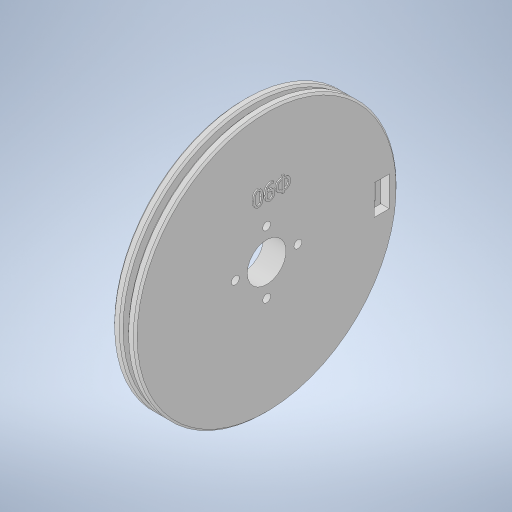
# Autodesk Inventor part: pully_shoulder2_90
Saved by Autodesk Inventor 2024 (Build 280153000, 153)
## iProperties
Created: 2025-06-10
Part Number: pully_shoulder2_90
Material: 一般
Document SubType Name: Modeling
Designer: HosodaLab2
Density: 1 g/cm^3
Appearance: 既定
Author: HosodaLab2
Autodesk Inventor part; units mm, degrees
ref_plane "YZ Plane" through (0, 0, 0) normal (1, 0, 0) x (0, 1, 0)
ref_plane "XZ Plane" through (0, 0, 0) normal (0, 1, 0) x (-1, 0, 0)
ref_plane "XY Plane" through (0, 0, 0) normal (0, 0, 1) x (1, 0, 0)
sketch "スケッチ1" plane through (0, 0, 0) normal (0, 1, 0) x (-1, 0, 0)
  circle A0 centre (0, 0) radius 45
  dimension "d0" = 90
  constraints: 1 centre point, 1 coincident
  measures "d0" diameter of A0
extrude "押し出し1" add sketch "スケッチ1" along normal blind 2.2
sketch "スケッチ2" plane through (0, 2.2, 0) normal (0, 1, 0) x (1, 0, 0)
  circle A0 centre (0, 0) radius 52.5
  line L0 (-4.0726, -27.1836) -> (5.4532, -27.1836) construction
  line L1 (5.4532, -27.1836) -> (5.4532, -31.1043) construction
  line L2 (5.4532, -31.1043) -> (-4.0726, -31.1043) construction
  line L3 (-4.0726, -31.1043) -> (-4.0726, -27.1836) construction
  dimension "d3" = 105
  constraints: 1 centre point, 1 coincident, 2 other
  measures "d3" diameter of A0
extrude "押し出し2" add sketch "スケッチ2" along normal blind 3.4
chamfer "面取り1" distance 0.75 angle 45 1 edges at (-52.5, 2.2, 0)
chamfer "面取り2" distance 0.75 angle 45 1 edges at (-52.5, 5.6, 0)
sketch "スケッチ3" plane through (0, 0, 0) normal (0, -1, 0) x (1, 0, 0)
  circle A0 centre (0, 0) radius 52.5
  dimension "d12" = 105
  constraints: 1 centre point, 1 coincident
  measures "d12" diameter of A0
extrude "押し出し3" add sketch "スケッチ3" along normal blind 3.4
chamfer "面取り3" distance 0.75 angle 45 1 edges at (-52.5, 0, 0)
chamfer "面取り4" distance 0.75 angle 45 1 edges at (-52.5, -3.4, 0)
sketch "スケッチ6" plane through (0, 5.6, 0) normal (0, 1, 0) x (1, 0, 0)
  circle A0 centre (0, 0) radius 7.65
  line L0 (0, 7.65) -> (46.8799, 7.65)
  circle A1 centre (0, 0) radius 47.5 projected
  line L1 (0, -7.65) -> (46.8799, -7.65)
  dimension "d39" = 15.3
  constraints: 4 end point, 4 point on circle, 1 centre point, 1 coincident, 1 horizontal, 1 parallel, 1 tangent
  measures "d39" diameter of A0
extrude "押し出し5" [suppressed]
chamfer "面取り7" [suppressed]
chamfer "面取り8" [suppressed]
chamfer "面取り9" [suppressed]
sketch "スケッチ7" plane through (0, 5.6, 0) normal (0, 1, 0) x (1, 0, 0)
  line L0 (-9.3358, -20.9354) -> (21.308, -20.9354) construction
  line L1 (21.308, -20.9354) -> (21.308, -27.5341) construction
  line L2 (21.308, -27.5341) -> (-9.3358, -27.5341) construction
  line L3 (-9.3358, -27.5341) -> (-9.3358, -20.9354) construction
  spline S0 degree 2 poles (-5.7914, -21.6571) (-5.2131, -21.667) (-4.2541, -22.0526) (-3.9377, -22.3739) knots 0 0 0 1 2 2 2
  spline S1 degree 2 poles (-3.9377, -22.3739) (-3.646, -22.6754) (-3.3247, -23.5207) (-3.3247, -24.0645) knots 0 0 0 1 2 2 2
  spline S2 degree 2 poles (-3.3247, -24.0645) (-3.3247, -24.633) (-3.6708, -25.5079) (-3.9772, -25.8045) knots 0 0 0 1 2 2 2
  spline S3 degree 2 poles (-3.9772, -25.8045) (-4.3084, -26.1308) (-5.2773, -26.4916) (-5.7914, -26.5015) knots 0 0 0 1 2 2 2
  line L4 (-5.7914, -26.5015) -> (-5.7914, -27.2084)
  line L5 (-5.7914, -27.2084) -> (-6.6021, -27.2084)
  line L6 (-6.6021, -27.2084) -> (-6.6021, -26.5015)
  spline S4 degree 2 poles (-6.6021, -26.5015) (-7.1162, -26.4867) (-8.0802, -26.1506) (-8.4213, -25.8144) knots 0 0 0 1 2 2 2
  spline S5 degree 2 poles (-8.4213, -25.8144) (-8.7277, -25.5129) (-9.0688, -24.628) (-9.0688, -24.0645) knots 0 0 0 1 2 2 2
  spline S6 degree 2 poles (-9.0688, -24.0645) (-9.0688, -23.5306) (-8.7426, -22.6853) (-8.446, -22.3788) knots 0 0 0 1 2 2 2
  spline S7 degree 2 poles (-8.446, -22.3788) (-8.1296, -22.0526) (-7.1805, -21.672) (-6.6021, -21.6571) knots 0 0 0 1 2 2 2
  line L7 (-6.6021, -21.6571) -> (-6.6021, -21.0096)
  line L8 (-6.6021, -21.0096) -> (-5.7914, -21.0096)
  line L9 (-5.7914, -21.0096) -> (-5.7914, -21.6571)
  spline S8 degree 2 poles (-5.7914, -25.8886) (-5.4207, -25.8787) (-4.8473, -25.6562) (-4.6594, -25.4684) knots 0 0 0 1 2 2 2
  spline S9 degree 2 poles (-4.6594, -25.4684) (-4.4073, -25.2212) (-4.17, -24.5143) (-4.17, -24.0299) knots 0 0 0 1 2 2 2
  spline S10 degree 2 poles (-4.17, -24.0299) (-4.17, -23.6245) (-4.3974, -22.9572) (-4.6248, -22.7249) knots 0 0 0 1 2 2 2
  spline S11 degree 2 poles (-4.6248, -22.7249) (-4.8374, -22.5024) (-5.4009, -22.2899) (-5.7914, -22.28) knots 0 0 0 1 2 2 2
  line L10 (-5.7914, -22.28) -> (-5.7914, -25.8886)
  spline S12 degree 2 poles (-6.6021, -22.28) (-6.9926, -22.2849) (-7.5562, -22.5074) (-7.7687, -22.7249) knots 0 0 0 1 2 2 2
  spline S13 degree 2 poles (-7.7687, -22.7249) (-7.9961, -22.9523) (-8.2235, -23.6344) (-8.2235, -24.0299) knots 0 0 0 1 2 2 2
  spline S14 degree 2 poles (-8.2235, -24.0299) (-8.2235, -24.5143) (-7.9862, -25.2262) (-7.7341, -25.4684) knots 0 0 0 1 2 2 2
  spline S15 degree 2 poles (-7.7341, -25.4684) (-7.5463, -25.6463) (-6.9729, -25.8836) (-6.6021, -25.8886) knots 0 0 0 1 2 2 2
  line L11 (-6.6021, -25.8886) -> (-6.6021, -22.28)
  spline S16 degree 2 poles (-2.781, -23.0412) (-2.781, -22.5716) (-2.4745, -21.7906) (-2.2076, -21.5088) knots 0 0 0 1 2 2 2
  spline S17 degree 2 poles (-2.2076, -21.5088) (-1.9555, -21.2369) (-1.2189, -20.9354) (-0.8432, -20.9354) knots 0 0 0 1 2 2 2
  spline S18 degree 2 poles (-0.8432, -20.9354) (-0.423, -20.9354) (0.2591, -21.2172) (0.5112, -21.4841) knots 0 0 0 1 2 2 2
  spline S19 degree 2 poles (0.5112, -21.4841) (0.8276, -21.8202) (1.1736, -22.9078) (1.1736, -23.7432) knots 0 0 0 1 2 2 2
  spline S20 degree 2 poles (1.1736, -23.7432) (1.1736, -24.4995) (0.8326, -25.854) (0.5014, -26.3038) knots 0 0 0 1 2 2 2
  spline S21 degree 2 poles (0.5014, -26.3038) (0.1504, -26.7784) (-0.8383, -27.2776) (-1.56, -27.2776) knots 0 0 0 1 2 2 2
  spline S22 degree 2 poles (-1.56, -27.2776) (-1.7231, -27.2776) (-2.0939, -27.243) (-2.252, -27.1936) knots 0 0 0 1 2 2 2
  line L12 (-2.252, -27.1936) -> (-2.252, -26.4076)
  line L13 (-2.252, -26.4076) -> (-2.2125, -26.4076)
  spline S23 degree 2 poles (-2.2125, -26.4076) (-2.1087, -26.4669) (-1.6737, -26.5707) (-1.4512, -26.5707) knots 0 0 0 1 2 2 2
  spline S24 degree 2 poles (-1.4512, -26.5707) (-0.6504, -26.5707) (0.2641, -25.5129) (0.3283, -24.5341) knots 0 0 0 1 2 2 2
  spline S25 degree 2 poles (0.3283, -24.5341) (0.0021, -24.7566) (-0.5911, -24.9592) (-0.9421, -24.9592) knots 0 0 0 1 2 2 2
  spline S26 degree 2 poles (-0.9421, -24.9592) (-1.2782, -24.9592) (-1.8368, -24.8109) (-2.1186, -24.5984) knots 0 0 0 1 2 2 2
  spline S27 degree 2 poles (-2.1186, -24.5984) (-2.4448, -24.3463) (-2.781, -23.5801) (-2.781, -23.0412) knots 0 0 0 1 2 2 2
  spline S28 degree 2 poles (0.3481, -23.5603) (0.3481, -22.9424) (0.1207, -22.1613) (-0.0819, -21.9488) knots 0 0 0 1 2 2 2
  spline S29 degree 2 poles (-0.0819, -21.9488) (-0.2599, -21.751) (-0.6307, -21.6027) (-0.8482, -21.6027) knots 0 0 0 1 2 2 2
  spline S30 degree 2 poles (-0.8482, -21.6027) (-1.3524, -21.6027) (-1.9505, -22.3245) (-1.9505, -23.0066) knots 0 0 0 1 2 2 2
  spline S31 degree 2 poles (-1.9505, -23.0066) (-1.9505, -23.3922) (-1.7528, -23.8915) (-1.5353, -24.0694) knots 0 0 0 1 2 2 2
  spline S32 degree 2 poles (-1.5353, -24.0694) (-1.3771, -24.198) (-0.9866, -24.282) (-0.7592, -24.282) knots 0 0 0 1 2 2 2
  spline S33 degree 2 poles (-0.7592, -24.282) (-0.4972, -24.282) (0.1059, -24.0991) (0.3333, -23.9459) knots 0 0 0 1 2 2 2
  spline S34 degree 2 poles (0.3333, -23.9459) (0.3382, -23.8865) (0.3481, -23.6839) (0.3481, -23.5603) knots 0 0 0 1 2 2 2
  spline S35 degree 2 poles (5.761, -24.109) (5.761, -25.7502) (4.8069, -27.2875) (3.8134, -27.2875) knots 0 0 0 1 2 2 2
  spline S36 degree 2 poles (3.8134, -27.2875) (2.8049, -27.2875) (1.8608, -25.7205) (1.8608, -24.1139) knots 0 0 0 1 2 2 2
  spline S37 degree 2 poles (1.8608, -24.1139) (1.8608, -22.4629) (2.8148, -20.9354) (3.8134, -20.9354) knots 0 0 0 1 2 2 2
  spline S38 degree 2 poles (3.8134, -20.9354) (4.8168, -20.9354) (5.761, -22.5173) (5.761, -24.109) knots 0 0 0 1 2 2 2
  spline S39 degree 2 poles (4.713, -25.9677) (4.8317, -25.6661) (4.9305, -24.7368) (4.9305, -24.109) knots 0 0 0 1 2 2 2
  spline S40 degree 2 poles (4.9305, -24.109) (4.9305, -23.4812) (4.8317, -22.5568) (4.7081, -22.2454) knots 0 0 0 1 2 2 2
  spline S41 degree 2 poles (4.7081, -22.2454) (4.5845, -21.9339) (4.1544, -21.6126) (3.8134, -21.6126) knots 0 0 0 1 2 2 2
  spline S42 degree 2 poles (3.8134, -21.6126) (3.4723, -21.6126) (3.0323, -21.9339) (2.9038, -22.2553) knots 0 0 0 1 2 2 2
  spline S43 degree 2 poles (2.9038, -22.2553) (2.7802, -22.5667) (2.6912, -23.5158) (2.6912, -24.1139) knots 0 0 0 1 2 2 2
  spline S44 degree 2 poles (2.6912, -24.1139) (2.6912, -24.7566) (2.7703, -25.6167) (2.8988, -25.9528) knots 0 0 0 1 2 2 2
  spline S45 degree 2 poles (2.8988, -25.9528) (3.0175, -26.2692) (3.4574, -26.6103) (3.8134, -26.6103) knots 0 0 0 1 2 2 2
  spline S46 degree 2 poles (3.8134, -26.6103) (4.1495, -26.6103) (4.5894, -26.289) (4.713, -25.9677) knots 0 0 0 1 2 2 2
  point P0 (0, 0)
  constraints: 2 other
extrude "押し出し6" add sketch "スケッチ7" along normal blind 0.5
sketch "スケッチ8" plane through (0, 5.6, 0) normal (0, 1, 0) x (1, 0, 0)
  line L0 (-43, 6) -> (-49, 6)
  line L1 (-49, 6) -> (-49, -6)
  line L2 (-49, -6) -> (-43, -6)
  line L3 (-43, -6) -> (-43, 6)
  arc A0 (-45, 0) -> (-45, 0) centre (0, 0) ccw projected
  point P0 (-46, -6)
  point P1 (-46, 6)
  dimension "d53" = 12
  dimension "d54" = 6
  dimension "d55" = 43
  constraints: 8 end point, 2 midpoint, 2 parallel, 1 horizontal, 1 perpendicular
  measures "d53" distance of point (-46, -6) point (-46, 6)
  measures "d54" distance between parallel lines of L1 L3
  measures "d55" distance from line of point (0, 0) L3
extrude "押し出し7" cut sketch "スケッチ8" against normal blind 7.5 contours L3 L2 A0 L0 | A0 L2 L1 L0 picked at (-43.6518, -0.6684)
sketch "スケッチ9" plane through (0, 5.6, 0) normal (0, 1, 0) x (1, 0, 0)
  point P0 (0, 0)
  point P1 (0, 0)
  constraints: 1 coincident
hole "穴2" at (0, 5.6, 0) direction (0, -1, 0) diameter 15.5 end through all
sketch "スケッチ10" plane through (0, 5.6, 0) normal (0, 1, 0) x (1, 0, 0)
  circle A0 centre (0, 0) radius 12.5 construction
  point P0 (0, -12.5)
  point P1 (12.5, 0)
  point P2 (0, 12.5)
  point P3 (-12.5, 0)
  dimension "d67" = 25
  dimension "d81" = 360
  constraints: 1 coincident, 1 vertical alignment, 7 other
hole "穴3" at (0, 5.6, 12.5) at (-12.5, 5.6, 0) at (0, 5.6, -12.5) at (12.5, 5.6, 0) direction (0, -1, 0) diameter 3.2 end through all
